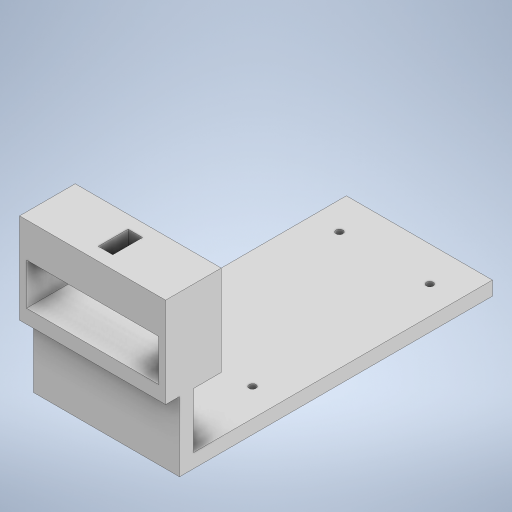
# Autodesk Inventor part: base
Saved by Autodesk Inventor 2023 (Build 270158000, 158)
## iProperties
Created: 2022-07-03
Part Number: base
Material: Genérico
Document SubType Name: Modeling
Designer: inigo
Density: 1 g/cm^3
Appearance: Valor por defecto
Author: inigo
Autodesk Inventor part; units mm, degrees
ref_plane "YZ Plane" through (0, 0, 0) normal (1, 0, 0) x (0, 1, 0)
ref_plane "XZ Plane" through (0, 0, 0) normal (0, 1, 0) x (-1, 0, 0)
ref_plane "XY Plane" through (0, 0, 0) normal (0, 0, 1) x (1, 0, 0)
sketch "Boceto1" plane through (0, 0, 0) normal (1, 0, 0) x (0, 1, 0)
  line L0 (10, 225) -> (-10, 225)
  line L1 (-10, 225) -> (-10, -225)
  line L2 (-10, -225) -> (10, -225)
  line L3 (10, -225) -> (10, 225)
  line L4 (10, 225) -> (-10, -225) construction
  line L5 (-10, 225) -> (10, -225) construction
  point P0 (0, 0)
  dimension "d0" = 20
  dimension "d1" = 450
  constraints: 12 end point, 2 midpoint, 2 parallel, 1 horizontal, 1 perpendicular
  measures "d0" distance of L2.end L1.end
  measures "d1" distance of L1.end L0.end
extrude "Extrusión1" add sketch "Boceto1" along normal blind 210
sketch "Boceto2" plane through (0, 10, 225) normal (0, 1, 0) x (1, 0, 0)
  line L0 (0, 0) -> (0, 450) projected
  line L1 (210, 0) -> (210, 450) projected
  line L2 (0, 0) -> (210, 0)
  line L3 (210, 0) -> (210, 20)
  line L4 (210, 20) -> (0, 20)
  line L5 (0, 20) -> (0, 0)
  point P0 (0, 225)
  dimension "d4" = 20
  constraints: 8 end point, 2 parallel, 1 horizontal, 1 perpendicular, 1 point on line
  measures "d4" distance of L3.end L2.end
extrude "Extrusión2" add sketch "Boceto2" along normal blind 80
sketch "Boceto3" plane through (0, 90, 225) normal (0, 1, 0) x (1, 0, 0)
  line L0 (0, 0) -> (210, 0) projected
  line L1 (0, 0) -> (210, 0)
  line L2 (210, 0) -> (210, -20)
  line L3 (210, -20) -> (0, -20)
  line L4 (0, -20) -> (0, 0)
  line L5 (0, 0) -> (210, 0)
  line L6 (210, 0) -> (210, 60)
  line L7 (210, 60) -> (0, 60)
  line L8 (0, 60) -> (0, 0)
  point P0 (0, 225)
  dimension "d7" = 20
  dimension "d8" = 210
  dimension "d9" = 60
  constraints: 16 end point, 4 parallel, 2 horizontal, 2 perpendicular
  measures "d7" distance of L1.end L2.end
  measures "d8" distance of L7.end L6.end
  measures "d9" distance of L6.end L5.end
extrude "Extrusión3" add sketch "Boceto3" along normal blind 130
sketch "Boceto4" plane through (0, 90, 245) normal (0, 0, 1) x (1, 0, 0)
  line L0 (10, 80) -> (200, 80)
  line L1 (200, 80) -> (200, 20)
  line L2 (200, 20) -> (10, 20)
  line L3 (10, 20) -> (10, 80)
  point P0 (0, -90)
  point P1 (0, 130)
  point P2 (210, 0)
  dimension "d12" = 190
  dimension "d13" = 60
  constraints: 8 end point, 2 parallel, 1 horizontal, 1 perpendicular
  measures "d12" distance of L1.end L2.end
  measures "d13" distance of L0.end L1.end
extrude "Extrusión4" cut sketch "Boceto4" against normal blind 60
sketch "Boceto5" plane through (0, 220, 225) normal (0, 1, 0) x (1, 0, 0)
  line L0 (94.5, -1.5) -> (115.5, -1.5)
  line L1 (115.5, -1.5) -> (115.5, 41.5)
  line L2 (115.5, 41.5) -> (94.5, 41.5)
  line L3 (94.5, 41.5) -> (94.5, -1.5)
  line L4 (94.5, -1.5) -> (115.5, 41.5) construction
  line L5 (115.5, -1.5) -> (94.5, 41.5) construction
  point P0 (0, 225)
  point P1 (105, 20)
  dimension "d18" = 21
  dimension "d19" = 43
  constraints: 12 end point, 2 midpoint, 2 parallel, 1 horizontal, 1 perpendicular
  measures "d18" distance of L2.end L1.end
  measures "d19" distance of L1.end L0.end
extrude "Extrusión5" cut sketch "Boceto5" against normal blind 43
sketch "Boceto6" plane through (0, 10, -225) normal (0, 1, 0) x (1, 0, 0)
  circle A0 centre (40, -305) radius 5
  circle A1 centre (40, -50) radius 5
  circle A2 centre (170, -305) radius 5
  circle A3 centre (170, -50) radius 5
  line L0 (0, -470) -> (210, -470) projected
  line L1 (0, 0) -> (210, 0) projected
  line L2 (0, 0) -> (0, -430) projected
  line L3 (210, 0) -> (210, -430) projected
  point P0 (0, -225)
  dimension "d23" = 10
  dimension "d24" = 10
  dimension "d25" = 10
  dimension "d26" = 10
  dimension "d27" = 165
  dimension "d28" = 50
  dimension "d29" = 50
  dimension "d30" = 165
  dimension "d31" = 40
  dimension "d32" = 40
  dimension "d33" = 40
  dimension "d34" = 40
  constraints: 4 centre point
  measures "d23" diameter of A0
  measures "d24" diameter of A1
  measures "d25" diameter of A2
  measures "d26" diameter of A3
  measures "d27" distance from line of L0 A0.centre
  measures "d28" distance from line of L1 A1.centre
  measures "d29" distance from line of L1 A3.centre
  measures "d30" distance from line of L0 A2.centre
  measures "d31" distance from line of L2 A0.centre
  measures "d32" distance from line of L2 A1.centre
  measures "d33" distance from line of L3 A3.centre
  measures "d34" distance from line of L3 A2.centre
extrude "Extrusión6" cut sketch "Boceto6" against normal blind 43
